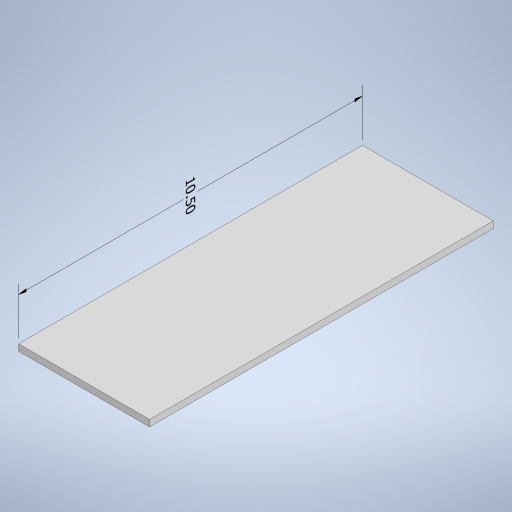
# Autodesk Inventor part: Top
Saved by Autodesk Inventor 2024.3 (Build 283343010, 343A)
## iProperties
Created: 2025-04-09
Part Number: Top
Material: Generic
Document SubType Name: Modeling
Designer: Vincent Larson
Density: 1 g/cm^3
Appearance: Default
Author: Vincent Larson
Autodesk Inventor part; units mm, degrees
ref_plane "YZ Plane" through (0, 0, 0) normal (1, 0, 0) x (0, 1, 0)
ref_plane "XZ Plane" through (0, 0, 0) normal (0, 1, 0) x (-1, 0, 0)
ref_plane "XY Plane" through (0, 0, 0) normal (0, 0, 1) x (1, 0, 0)
sketch "Sketch1" plane through (0, 0, 0) normal (0, 1, 0) x (-1, 0, 0)
  line L0 (50.8, 133.35) -> (-50.8, 133.35)
  line L1 (-50.8, 133.35) -> (-50.8, -133.35)
  line L2 (-50.8, -133.35) -> (50.8, -133.35)
  line L3 (50.8, -133.35) -> (50.8, 133.35)
  line L4 (50.8, 133.35) -> (-50.8, -133.35) construction
  line L5 (-50.8, 133.35) -> (50.8, -133.35) construction
  point P0 (0, 0)
  dimension "d0" = 101.6
  dimension "d1" = 266.7
  constraints: 12 end point, 2 midpoint, 2 parallel, 1 horizontal, 1 perpendicular
  measures "d0" distance of L2.end L1.end
  measures "d1" distance of L1.end L0.end
extrude "Extrusion1" add sketch "Sketch1" along normal blind 5.08
body "Solid1"
